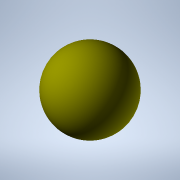
# Autodesk Inventor part: 22.225-52-34.1-15-ybrg1-507.938-39.04-b
Saved by Autodesk Inventor 2021 (Build 250183000, 183)
## iProperties
Created: 2025-11-05
Part Number: 22.225-52-34.1-15-ybrg1-507.938-39.04-b
Material: Generic
Catalog Web Link: www.3dfindit.com
Description: ayp_001_hc_hh_hy-ayl_001_hp_ball-Y-bearings
Vendor: SKF
Document SubType Name: Modeling
Designer: psAdmin
Manufacturer: SKF
Mass: 0.261898 g
Surface Area: 1.97958 cm^2
Volume: 0.261898 cm^3
Density: 1 g/cm^3
Appearance: PSOLRGB-255-255-0
Category: PARTsolutions
Company: SKF
Title: 22.225-52-34.1-15-ybrg1-507.938-39.04-b
Author: Cadenas PARTsolutions
Comments: Y-bearings
PSOL_IDENT_0: {$CADENAS_DATA/23d-libs/skf/bearings_units_and_housings/bearing_units/ball_bearing_units/y-units/y-b
PSOL_IDENT_1: earing_plummer_block_units_parts/ayp_001_hc_hh_hy-ayl_001_hp_ball.prj},246 {VTYP=3D},{NB=22.225-52-3
PSOL_IDENT_2: 4.1-15-ybrg1-507.938-39.04-b},{LINA=22.225-52-34.1-15-ybrg1-507.938-39.04-b},{NN=ayp_001_hc_hh_hy-ay
PSOL_IDENT_3: l_001_hp_ball},{DATE=09.09.2022 05:06:20},{GEOMDATE=05.09.2022 09:08:52},{VERSION=},{LINEID=3080},{W
PSOL_IDENT_4: BVAR=},{WBNUMERIC=}  {NB=22.225-52-34.1-15-ybrg1-507.938-39.04-b},{LINA=22.225-52-34.1-15-ybrg1-507.
PSOL_IDENT_5: 938-39.04-b},{KT=DUMMY},{DD=22.2250},{D=52},{B=34.100},{C=15.000},{PITCH=39.040},{DW=7.938},{FO=IEC_
PSOL_IDENT_6: BBY_006},{DESIGN=ybrg1},{X=0},{PN=50}
NB: 22.225-52-34.1-15-ybrg1-507.938-39.04-b
NN: ayp_001_hc_hh_hy-ayl_001_hp_ball
NT: Y-bearings
NBSYN: $DD.-$D.-$B.-$C.-$DESIGN.-$PN.$DW.-$PITCH.-b
LINA: 22.225-52-34.1-15-ybrg1-507.938-39.04-b
CATALOG: SKF
DD: 22.225
D: 52
B: 34.1
C: 15
PITCH: 39.04
DW: 7.938
FO: IEC_BBY_006
DESIGN: ybrg1
PN: 50
SUPPLIER: SKF
ARTICLENO: 22.225-52-34.1-15-ybrg1-507.938-39.04-b
BOMINFO: 22.225-52-34.1-15-ybrg1-507.938-39.04-b
CREATOR: CADENAS GmbH
Autodesk Inventor part; units mm, degrees
sketch "Sketch_1" plane through (0, 0, 0) normal (0, 0, 1) x (1, 0, 0)
  line L0 (3.969, 19.52) -> (-3.969, 19.52)
  arc A0 (3.969, 19.52) -> (-3.969, 19.52) centre (0, 19.52) ccw
  line L1 (3.969, 19.52) -> (-3.969, 19.52)
  constraints: 4 end point, 2 point on circle, 1 centre point
revolve "Revolution1" add sketch "Sketch_1" angle 360 about axis through (3.969, 19.52, 0) along (1, 0, 0)
ref_plane "ball_XY" through (0, 19.52, 0) normal (1, 0, 0) x (0, 0, -1)
ref_plane "ball_YZ" through (0, 19.52, 0) normal (0, 0, -1) x (0, 1, 0)
ref_plane "ball_ZX" through (0, 19.52, 0) normal (0, 1, 0) x (1, 0, 0)
body "Solid1"
